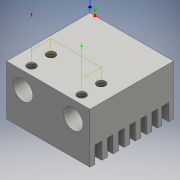
# Autodesk Inventor part: nozzel heat sink
Saved by Autodesk Inventor 2016 SP1 (Build 200210100, 210)
## iProperties
Created: 2016-03-06
Part Number: nozzel heat sink
Material: Generic
Document SubType Name: Modeling
Designer: roduino
Density: 1 g/cm^3
Appearance: Default
Author: roduino
Autodesk Inventor part; units mm, degrees
ref_plane "YZ Plane" through (0, 0, 0) normal (1, 0, 0) x (0, 1, 0)
ref_plane "XZ Plane" through (0, 0, 0) normal (0, 1, 0) x (-1, 0, 0)
ref_plane "XY Plane" through (0, 0, 0) normal (0, 0, 1) x (1, 0, 0)
sketch "Sketch1" plane through (0, 0, 0) normal (0, 0, 1) x (1, 0, 0)
  line L0 (-15, 15) -> (15, 15)
  line L1 (15, 15) -> (15, -15)
  line L2 (15, -15) -> (-15, -15)
  line L3 (-15, -15) -> (-15, 15)
  point P0 (0, 0)
  dimension "d0" = 30
  dimension "d1" = 30
  dimension "d2" = 15
  dimension "d3" = 15
  constraints: 8 end point, 2 parallel, 1 horizontal, 1 perpendicular
  measures "d0" distance of L0.start L0.end
  measures "d1" distance of L2.end L0.start
  measures "d2" distance from line of point (0, 0) L0
  measures "d3" distance from line of point (0, 0) L3
extrude "Extrusion1" add sketch "Sketch1" along normal blind 18
sketch "Sketch2" plane through (-15, 15, 0) normal (0, 1, 0) x (1, 0, 0)
  circle A0 centre (6.5, -3) radius 1.5
  circle A1 centre (23.5, -3) radius 1.5
  circle A2 centre (15, -15) radius 1.5
  circle A3 centre (6, -12) radius 2.5
  circle A4 centre (24, -12) radius 2.5
  line L0 (0, 0) -> (30, 0) projected
  line L1 (15, 0) -> (15, -28.1045) construction
  line L2 (30, -18) -> (0, -18) construction
  line L3 (6, -12) -> (24, -12) construction
  dimension "d6" = 3
  dimension "d7" = 3
  dimension "d8" = 3
  dimension "d9" = 5
  dimension "d10" = 5
  dimension "d11" = 17
  dimension "d12" = 3
  dimension "d13" = 3
  dimension "d14" = 8.5
  dimension "d15" = 18
  dimension "d16" = 9
  dimension "d17" = 3
  dimension "d18" = 6
  dimension "d19" = 6
  dimension "d20" = 0
  dimension "d51" = 3
  dimension "d52" = 9
  constraints: 5 centre point, 4 end point, 1 vertical
  measures "d6" diameter of A0
  measures "d7" diameter of A1
  measures "d8" diameter of A2
  measures "d9" diameter of A3
  measures "d10" diameter of A4
  measures "d11" distance of A1.centre A0.centre
  measures "d12" distance from line of L0 A0.centre
  measures "d13" distance from line of L0 A1.centre
  measures "d14" horizontal distance of L1.start A0.centre
  measures "d15" distance of L3.end L3.start
  measures "d16" distance from line of L1 L3.start
  measures "d17" distance from line of L2 A2.centre
  measures "d18" distance from line of L2 L3.start
  measures "d19" distance from line of L2 L3.end
  measures "d20" distance from line of L1 A2.centre
  measures "d51" distance from line of L3 A2.centre
  measures "d52" distance from line of L3 A0.centre
extrude "Extrusion2" cut sketch "Sketch2" against normal blind 10
thread "Thread3" size "M3x0.5" class "6H" standard "ANSI Metric M Profile" full length
thread "Thread4" size "M3x0.5" class "6H" standard "ANSI Metric M Profile" full length
thread "Thread5" size "M3x0.5" class "6H" standard "ANSI Metric M Profile" full length
sketch "Sketch3" plane through (-9, 5, 12) normal (0, 1, 0) x (1, 0, 0)
  circle A0 centre (0, 0) radius 1
  point P0 (9, 12)
  dimension "d23" = 2
  constraints: 1 centre point
  measures "d23" diameter of A0
extrude "Extrusion3" cut sketch "Sketch3" against normal through all
sketch "Sketch4" plane through (9, 5, 12) normal (0, 1, 0) x (1, 0, 0)
  circle A0 centre (0, 0) radius 1
  point P0 (-9, 12)
  dimension "d26" = 2
  constraints: 1 centre point
  measures "d26" diameter of A0
extrude "Extrusion4" cut sketch "Sketch4" against normal through all
sketch "Sketch5" plane through (-15, -15, 0) normal (0, -1, 0) x (1, 0, 0)
  circle A0 centre (6, 12) radius 1 projected
  circle A1 centre (6, 12) radius 3.5
  circle A2 centre (24, 12) radius 1 projected
  circle A3 centre (24, 12) radius 3.5
  point P0 (15, 0)
  dimension "d29" = 7
  dimension "d30" = 7
  constraints: 2 centre point, 2 coincident
  measures "d29" diameter of A1
  measures "d30" diameter of A3
extrude "Extrusion5" cut sketch "Sketch5" against normal blind 15
sketch "Sketch6" plane through (0, 0, 0) normal (0, 0, -1) x (-1, 0, 0)
  line L0 (15, 15) -> (15, -15) projected
  line L1 (-15, -13.25) -> (15, -13.25)
  line L2 (15, -13.25) -> (15, -10.75)
  line L3 (15, -10.75) -> (-15, -10.75)
  line L4 (-15, -10.75) -> (-15, -13.25)
  line L5 (-15, -15) -> (15, -15) projected
  line L6 (-15, 10.75) -> (15, 10.75)
  line L7 (15, 10.75) -> (15, 13.25)
  line L8 (15, 13.25) -> (-15, 13.25)
  line L9 (-15, 13.25) -> (-15, 10.75)
  line L10 (15, 15) -> (-15, 15) projected
  line L11 (-15, -8.75) -> (15, -8.75)
  line L12 (15, -8.75) -> (15, -6.75)
  line L13 (15, -6.75) -> (-15, -6.75)
  line L14 (-15, -6.75) -> (-15, -8.75)
  line L15 (15, -2.75) -> (-15, -2.75)
  line L16 (-15, -2.75) -> (-15, -4.75)
  line L17 (-15, -4.75) -> (15, -4.75)
  line L18 (15, -4.75) -> (15, -2.75)
  line L19 (15, 1.25) -> (-15, 1.25)
  line L20 (-15, 1.25) -> (-15, -0.75)
  line L21 (-15, -0.75) -> (15, -0.75)
  line L22 (15, -0.75) -> (15, 1.25)
  line L23 (15, 5.25) -> (-15, 5.25)
  line L24 (-15, 5.25) -> (-15, 3.25)
  line L25 (-15, 3.25) -> (15, 3.25)
  line L26 (15, 3.25) -> (15, 5.25)
  line L27 (15, 9.25) -> (-15, 9.25)
  line L28 (-15, 9.25) -> (-15, 7.25)
  line L29 (-15, 7.25) -> (15, 7.25)
  line L30 (15, 7.25) -> (15, 9.25)
  point P0 (0, 0)
  dimension "d33" = 30
  dimension "d34" = 30
  dimension "d35" = 2.5
  dimension "d36" = 1.75
  dimension "d37" = 2.5
  dimension "d38" = 30
  dimension "d39" = 1.75
  dimension "d40" = 2
  dimension "d41" = 2
  dimension "d44" = 4
  constraints: 56 end point, 6 parallel, 3 horizontal, 3 perpendicular, 3 point on line, 1 vertical, 32 other
  measures "d33" distance of L5.start L0.end
  measures "d34" distance of L1.start L1.end
  measures "d35" distance between parallel lines of L3 L1
  measures "d36" distance between parallel lines of L5 L1
  measures "d37" distance of L8.end L6.start
  measures "d38" distance of L7.end L8.end
  measures "d39" distance between parallel lines of L10 L8
  measures "d40" distance of L13.end L11.start
  measures "d41" distance between parallel lines of L3 L11
  measures "d44" distance of L12.end L15.start
extrude "Extrusion6" cut sketch "Sketch6" against normal blind 6
thread "Thread1" size "M5x0.8" class "6H" standard "ANSI Metric M Profile" full length
thread "Thread2" size "M5x0.8" class "6H" standard "ANSI Metric M Profile" full length
sketch "Sketch7" plane through (0, 0, 18) normal (0, 0, 1) x (1, 0, 0)
  circle A0 centre (-9, -12) radius 1.5
  circle A1 centre (9, -12) radius 1.5
  circle A2 centre (9, -5) radius 1.5
  circle A3 centre (-9, -5) radius 1.5
  line L0 (-5.5, -15) -> (-12.5, -15) projected
  line L1 (-15, -15) -> (15, -15) projected
  point P0 (0, 0)
  dimension "d63" = 3
  dimension "d64" = 3
  dimension "d65" = 3
  dimension "d66" = 3
  dimension "d67" = 18
  dimension "d68" = 18
  dimension "d69" = 9
  dimension "d70" = 9
  dimension "d71" = 3
  dimension "d72" = 3
  dimension "d73" = 7
  dimension "d74" = 7
  constraints: 4 centre point
  measures "d63" diameter of A0
  measures "d64" diameter of A1
  measures "d65" diameter of A2
  measures "d66" diameter of A3
  measures "d67" distance of A2.centre A3.centre
  measures "d68" distance of A1.centre A0.centre
  measures "d69" horizontal distance of point (0, 0) A3.centre
  measures "d70" horizontal distance of point (0, 0) A0.centre
  measures "d71" distance from line of L0 A0.centre
  measures "d72" distance from line of L1 A1.centre
  measures "d73" distance of A0.centre A3.centre
  measures "d74" distance of A1.centre A2.centre
extrude "Extrusion7" cut sketch "Sketch7" against normal up to next
thread "Thread6" size "M3x0.5" class "6H" standard "ANSI Metric M Profile" full length
thread "Thread7" size "M3x0.5" class "6H" standard "ANSI Metric M Profile" full length
thread "Thread8" size "M3x0.5" class "6H" standard "ANSI Metric M Profile" full length
thread "Thread9" size "M3x0.5" class "6H" standard "ANSI Metric M Profile" full length
equation "\"d2\" = 0.5 * d1"
equation "\"d3\" = 0.5 * d0"
equation "\"d13\" = d12"
equation "\"d14\" = 0.5 * d11"
equation "\"d16\" = 0.5 * d15"
equation "\"d19\" = d18"
equation "\"d34\" = d33"
equation "\"d37\" = d35"
equation "\"d38\" = d33"
equation "\"d39\" = d36"
equation "\"d41\" = d40"
equation "\"d68\" = d67"
equation "\"d69\" = 0.5 * d67"
equation "\"d70\" = d69"
equation "\"d74\" = d73"
body "Solid1"
